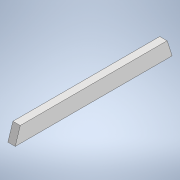
# Autodesk Inventor part: LegConnector_1
Saved by Autodesk Inventor 2022 (Build 260153000, 153)
## iProperties
Created: 2022-01-15
Part Number: LegConnector_1
Material: Generic
Document SubType Name: Modeling
Designer: dangl
Density: 1 g/cm^3
Appearance: Default
Author: dangl
Autodesk Inventor part; units mm, degrees
ref_plane "YZ Plane" through (0, 0, 0) normal (1, 0, 0) x (0, 1, 0)
ref_plane "XZ Plane" through (0, 0, 0) normal (0, 1, 0) x (-1, 0, 0)
ref_plane "XY Plane" through (0, 0, 0) normal (0, 0, 1) x (1, 0, 0)
sketch "Sketch1" plane through (0, 0, 0) normal (1, 0, 0) x (0, 1, 0)
  line L0 (-361.9542, 237.9953) -> (349.2458, 9.3298) projected
  line L1 (349.2458, 9.3298) -> (268.4937, 35.2933)
  line L2 (268.4937, 35.2933) -> (268.4937, -371.1067)
  line L3 (349.2458, 9.3298) -> (349.2458, -371.1067)
  line L4 (349.2458, -371.1067) -> (268.4937, -371.1067)
  line L5 (268.4937, -777.5067) -> (268.4937, -371.1067)
  line L6 (349.2458, -751.5433) -> (349.2458, -371.1067)
  line L7 (349.2458, -751.5433) -> (268.4937, -777.5067)
  point P0 (0, 0)
  dimension "d0" = 406.4
  dimension "d1" = 80.7521
  constraints: 14 end point, 2 symmetric about line, 2 vertical, 1 perpendicular, 1 point on line
  measures "d0" distance of L1.end L2.end
  measures "d1" distance from line of L0.end L2
extrude "Extrusion1" add sketch "Sketch1" along normal mid plane 38.1
body "Solid1"
